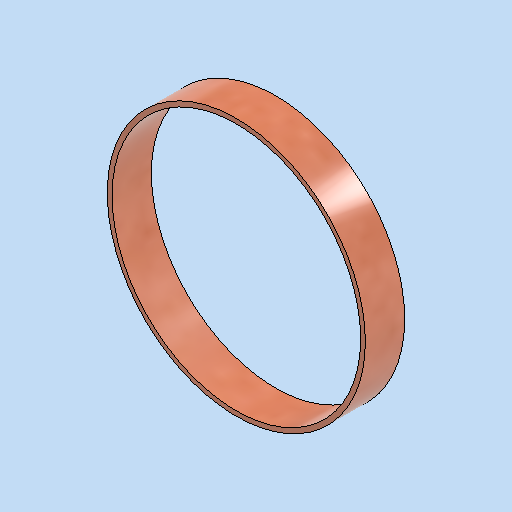
# Autodesk Inventor part: TouptekAdapterRing
Saved by Autodesk Inventor 2025 (Build 290162000, 162)
## iProperties
Created: 2025-02-20
Part Number: TouptekAdapterRing
Material: ABS Plastic
Document SubType Name: Modeling
Designer: kuzmin
Density: 1.06 g/cm^3
Appearance: Walnut - Natural Polished
Author: kuzmin
Autodesk Inventor part; units mm, degrees
ref_plane "YZ Plane" through (0, 0, 0) normal (1, 0, 0) x (0, 1, 0)
ref_plane "XZ Plane" through (0, 0, 0) normal (0, 1, 0) x (-1, 0, 0)
ref_plane "XY Plane" through (0, 0, 0) normal (0, 0, 1) x (1, 0, 0)
sketch "Sketch1" plane through (0, 0, 0) normal (0, 0, 1) x (1, 0, 0)
  circle A0 centre (0, 0) radius 15.8
  circle A1 centre (0, 0) radius 16.4
  dimension "d0" = 31.6
  dimension "d1" = 32.8
  constraints: 2 centre point, 2 coincident
  measures "d0" diameter of A0
  measures "d1" diameter of A1
extrude "Extrusion1" add sketch "Sketch1" along normal blind 5
equation "\"d0\" = inner"
equation "\"d1\" = outer"
equation "\"inner\" = 31.6"
equation "\"outer\" = 32.8"
body "Solid1"
